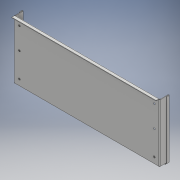
# Autodesk Inventor part: 4-2
Saved by Autodesk Inventor 2017 (Build 210142000, 142)
## iProperties
Part Number: 4-2
Material: 一般
Document SubType Name: 板金
Designer: Brian
Density: 1 g/cm^3
Sheet Metal Rule: 預設
Appearance: 預設
Mass: 286.375 g
Surface Area: 2901.47 cm^2
Volume: 286.375 cm^3
Author: Brian
Autodesk Inventor part; units mm, degrees
ref_plane "YZ Plane" through (0, 0, 0) normal (1, 0, 0) x (0, 1, 0)
ref_plane "XZ Plane" through (0, 0, 0) normal (0, 1, 0) x (-1, 0, 0)
ref_plane "XY Plane" through (0, 0, 0) normal (0, 0, 1) x (1, 0, 0)
sketch "草圖1" plane through (0, 0, 0) normal (0, 1, 0) x (-1, 0, 0)
  line L0 (0, 0) -> (-500, 0)
  line L1 (-500, 0) -> (-500, -200)
  line L2 (-500, -200) -> (0, -200)
  line L3 (0, -200) -> (0, 0)
  dimension "d0" = 200
  dimension "d1" = 500
  measures "d0" distance of L2.end L0.start
  measures "d1" distance of L1.end L2.end
extrude "平板1" add sketch "草圖1" against normal blind 2
sketch "草圖2" plane through (0, 0, 0) normal (0, 1, 0) x (1, 0, 0)
  line L0 (16, 180) -> (484, 180)
  line L1 (484, 180) -> (484, 20)
  line L2 (484, 20) -> (16, 20)
  line L3 (16, 20) -> (16, 180)
  line L4 (500, 200) -> (0, 200) projected
  line L5 (0, 200) -> (0, 0) projected
  line L6 (16, 95) -> (484, 95)
  dimension "d3" = 468
  dimension "d4" = 20
  dimension "d5" = 16
  dimension "d7" = 85
  dimension "d8" = 75
  constraints: 10 end point, 2 parallel, 2 perpendicular, 2 point on line, 1 horizontal
  measures "d3" distance of L0.start L0.end
  measures "d4" distance between parallel lines of L4 L0
  measures "d5" distance between parallel lines of L5 L3
  measures "d7" distance between parallel lines of L0 L6
  measures "d8" distance between parallel lines of L2 L6
hole "孔1" at (16, 0, -180) at (16, 0, -95) at (16, 0, -20) at (484, 0, -20) at (484, 0, -95) at (484, 0, -180) direction (0, -1, 0) diameter 6.5 depth 2 tip angle 118 countersink diameter 10.5 countersink angle 91
sketch "草圖3" plane through (500.74, 0.74, -200) normal (1, 0, 0) x (0, 1, 0)
  line L0 (0, 200) -> (0, 0)
  line L1 (0, 0) -> (29.26, 0)
  line L2 (29.26, 0) -> (29.26, 200)
  line L3 (29.26, 200) -> (0, 200)
  constraints: 6 end point, 1 horizontal, 1 perpendicular, 1 vertical
edge flange "凸緣1" height 30 angle 90 thickness 2 bend radius 0.74 thickness toward (1, 0, 0) relief tear relief width 2 relief depth 1 edges at (500, 0, -100) wall of the first edge with corners at (500.74, 0.74, 0) (500.74, 0.74, -200) (500.74, 30, -200) (500.74, 30, 0)
bend "折彎1"
corner "轉角1"
sketch "草圖4" plane through (0, 0.74, -200.74) normal (0, 0, -1) x (-1, 0, 0)
  line L0 (-500, 0) -> (0, 0)
  line L1 (0, 0) -> (0, 29.26)
  line L2 (0, 29.26) -> (-500, 29.26)
  line L3 (-500, 29.26) -> (-500, 0)
  constraints: 6 end point, 1 horizontal, 1 perpendicular, 1 vertical
edge flange "凸緣2" height 30 angle 90 thickness 2 bend radius 0.74 thickness toward (0, 0, -1) relief tear relief width 2 relief depth 1 edges at (250, 0, -200) wall of the first edge with corners at (500, 0.74, -200.74) (0, 0.74, -200.74) (0, 30, -200.74) (500, 30, -200.74)
bend "折彎2"
corner "轉角2"
sketch "草圖5" plane through (-0.74, 0.74, 0) normal (-1, 0, 0) x (0, -1, 0)
  line L0 (0, -200) -> (0, 0)
  line L1 (0, 0) -> (-29.26, 0)
  line L2 (-29.26, 0) -> (-29.26, -200)
  line L3 (-29.26, -200) -> (0, -200)
  constraints: 6 end point, 1 horizontal, 1 perpendicular, 1 vertical
edge flange "凸緣3" height 30 angle 90 thickness 2 bend radius 0.74 thickness toward (-1, 0, 0) relief tear relief width 2 relief depth 1 edges at (0, 0, -100) wall of the first edge with corners at (-0.74, 0.74, -200) (-0.74, 0.74, 0) (-0.74, 30, 0) (-0.74, 30, -200)
bend "折彎3"
corner "轉角3"
sketch "草圖6" plane through (0, -2.74, 0.74) normal (0, 0, 1) x (1, 0, 0)
  line L0 (500, 0) -> (0, 0)
  line L1 (0, 0) -> (0, -9.26)
  line L2 (0, -9.26) -> (500, -9.26)
  line L3 (500, -9.26) -> (500, 0)
  constraints: 6 end point, 1 horizontal, 1 perpendicular, 1 vertical
edge flange "凸緣4" height 10 angle 90 thickness 2 bend radius 0.74 thickness toward (0, 0, 1) relief tear relief width 2 relief depth 1 edges at (250, -2, 0) wall of the first edge with corners at (500, -2.74, 0.74) (0, -2.74, 0.74) (0, -12, 0.74) (500, -12, 0.74)
bend "折彎4"
corner "轉角4"
sketch "草圖7" plane through (502.74, 27.5, -200) normal (0, 0, -1) x (-1, 0, 0)
  line L0 (2, 0) -> (0, 0)
  arc A0 (0, 0) -> (-1, 0) centre (-0.5, 0) ccw
  line L1 (-1, 0) -> (-1, -7.5)
  line L2 (-1, -7.5) -> (-3, -7.5)
  line L3 (-3, -7.5) -> (-3, 0)
  arc A1 (2, 0) -> (-3, 0) centre (-0.5, 0) ccw
  constraints: 8 end point, 4 point on circle
hem "折邊1" sketch "草圖7" thickness 2 along (0, 0, 1) edges at (502.74, 30, -100)
sketch "草圖8" plane through (0, 27.5, -202.74) normal (-1, 0, 0) x (0, -1, 0)
  line L0 (0, 2) -> (0, 0)
  arc A0 (0, 0) -> (0, -1) centre (0, -0.5) ccw
  line L1 (0, -1) -> (7.5, -1)
  line L2 (7.5, -1) -> (7.5, -3)
  line L3 (7.5, -3) -> (0, -3)
  arc A1 (0, 2) -> (0, -3) centre (0, -0.5) ccw
  constraints: 8 end point, 4 point on circle
hem "折邊2" sketch "草圖8" thickness 2 along (1, 0, 0) edges at (250, 30, -202.74)
sketch "草圖9" plane through (-2.74, 27.5, 0) normal (0, 0, 1) x (1, 0, 0)
  line L0 (2, 0) -> (0, 0)
  arc A0 (0, 0) -> (-1, 0) centre (-0.5, 0) ccw
  line L1 (-1, 0) -> (-1, -7.5)
  line L2 (-1, -7.5) -> (-3, -7.5)
  line L3 (-3, -7.5) -> (-3, 0)
  arc A1 (2, 0) -> (-3, 0) centre (-0.5, 0) ccw
  constraints: 8 end point, 4 point on circle
hem "折邊3" sketch "草圖9" thickness 2 along (0, 0, -1) edges at (-2.74, 30, -100)
equation "\"d14\" = 厚度"
equation "\"d56\" = 折彎離隙寬度"
equation "\"d57\" = 折彎離隙深度"
equation "\"d58\" = 最小剩餘"
equation "\"d59\" = 折彎半徑"
equation "\"d61\" = 0.5 * 厚度"
equation "\"d62\" = 0.5 * d61"
equation "\"d63\" = 折彎離隙寬度"
equation "\"d64\" = 折彎離隙深度"
equation "\"d65\" = 最小剩餘"
equation "\"d66\" = 折彎半徑"
equation "\"d68\" = 0.5 * 厚度"
equation "\"d69\" = 0.5 * d68"
equation "\"d70\" = 折彎離隙寬度"
equation "\"d71\" = 折彎離隙深度"
equation "\"d72\" = 最小剩餘"
equation "\"d73\" = 折彎半徑"
equation "\"d75\" = 0.5 * 厚度"
equation "\"d76\" = 0.5 * d75"
equation "\"d16\" = 折彎離隙寬度"
equation "\"d17\" = 折彎離隙深度"
equation "\"d18\" = 最小剩餘"
equation "\"d19\" = 折彎半徑"
equation "\"d23\" = 轉角離隙大小"
equation "\"d24\" = 間隙大小"
equation "\"d25\" = Jacobi半徑大小"
equation "\"d26\" = 折彎離隙寬度"
equation "\"d27\" = 折彎離隙深度"
equation "\"d28\" = 最小剩餘"
equation "\"d29\" = 折彎半徑"
equation "\"d33\" = 轉角離隙大小"
equation "\"d34\" = 間隙大小"
equation "\"d35\" = Jacobi半徑大小"
equation "\"d36\" = 折彎離隙寬度"
equation "\"d37\" = 折彎離隙深度"
equation "\"d38\" = 最小剩餘"
equation "\"d39\" = 折彎半徑"
equation "\"d43\" = 轉角離隙大小"
equation "\"d44\" = 間隙大小"
equation "\"d45\" = Jacobi半徑大小"
equation "\"d46\" = 折彎離隙寬度"
equation "\"d47\" = 折彎離隙深度"
equation "\"d48\" = 最小剩餘"
equation "\"d49\" = 折彎半徑"
equation "\"d53\" = 轉角離隙大小"
equation "\"d54\" = 間隙大小"
equation "\"d55\" = Jacobi半徑大小"
equation "\"折彎半徑\" = 厚度"
equation "\"折彎離隙寬度\" = 厚度"
equation "\"折彎離隙深度\" = 0.5 * 厚度"
equation "\"轉角離隙大小\" = 4 * 厚度"
equation "\"最小剩餘\" = 2 * 厚度"
equation "\"轉移半徑\" = 折彎半徑"
equation "\"Jacobi半徑大小\" = 厚度"
equation "\"間隙大小\" = 厚度"
equation "\"d2\" = 折彎半徑"
equation "\"厚度\" = 2"
